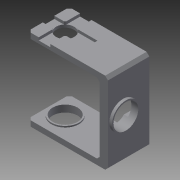
# Autodesk Inventor part: Enlace1
Saved by Autodesk Inventor 2015 (Build 190159000, 159)
## iProperties
Created: 2013-10-22
Part Number: Enlace1
Material: Genérico
Document SubType Name: Modeling
Designer: Gregorio
Density: 1 g/cm^3
Appearance: Valor por defecto
Author: Gregorio
Autodesk Inventor part; units mm, degrees
ref_plane "YZ Plane" through (0, 0, 0) normal (1, 0, 0) x (0, 1, 0)
ref_plane "XZ Plane" through (0, 0, 0) normal (0, 1, 0) x (-1, 0, 0)
ref_plane "XY Plane" through (0, 0, 0) normal (0, 0, 1) x (1, 0, 0)
sketch "Boceto1" plane through (0, 0, 0) normal (0, 1, 0) x (-1, 0, 0)
  line L0 (0, 0) -> (4, 0)
  line L1 (4, 0) -> (4, 58)
  line L2 (4, 58) -> (0, 58)
  line L3 (0, 58) -> (0, 0)
  line L4 (4, 58) -> (59, 58)
  line L5 (59, 58) -> (59, 54)
  line L6 (59, 54) -> (4, 54)
  line L7 (4, 54) -> (4, 58)
  line L8 (4, 0) -> (59, 0)
  line L9 (59, 0) -> (59, 4)
  line L10 (59, 4) -> (4, 4)
  line L11 (4, 4) -> (4, 0)
  dimension "d4" = 58
  dimension "d5" = 55
  dimension "d6" = 4
  dimension "d7" = 55
  dimension "d8" = 4
  dimension "d54" = 4
  constraints: 24 end point, 6 parallel, 3 horizontal, 3 perpendicular
  measures "d4" distance of L0.end L1.end
  measures "d5" distance of L5.end L6.end
  measures "d6" distance of L4.end L5.end
  measures "d7" distance of L10.end L9.end
  measures "d8" distance of L9.end L8.end
  measures "d54" distance of L1.end L2.end
extrude "Extrusión1" add sketch "Boceto1" along normal blind 30
sketch "Boceto3" plane through (-59, 0, 4) normal (0, 0, 1) x (1, 0, 0)
  line L0 (0, 0) -> (0, 30) projected
  circle A0 centre (12, 15) radius 9
  point P0 (59, 0)
  point P1 (0, 15)
  dimension "d19" = 18
  dimension "d20" = 12
  constraints: 1 centre point, 1 horizontal alignment, 1 midpoint
  measures "d19" diameter of A0
  measures "d20" distance from line of L0 A0.centre
extrude "Extrusión2" cut sketch "Boceto3" against normal blind 8 and the other way blind 2
sketch "Boceto5" plane through (0, 0, 58) normal (1, 0, 0) x (0, 0, -1)
  circle A0 centre (29, 11) radius 9
  line L0 (0, 30) -> (58, 30) projected
  line L1 (0, 0) -> (58, 0) projected
  line L2 (58, 0) -> (58, 30) projected
  line L3 (0, 0) -> (0, 30) projected
  point P0 (29, 30)
  point P1 (29, 30)
  dimension "d28" = 18
  dimension "d73" = 11
  constraints: 2 midpoint, 2 vertical alignment, 1 centre point
  measures "d28" diameter of A0
  measures "d73" distance from line of L1 A0.centre
extrude "Extrusión4" cut sketch "Boceto5" against normal blind 20 contours A0
sketch "Boceto6" plane through (-4, 0, 4) normal (-1, 0, 0) x (0, 0, 1)
  circle A0 centre (25, 11) radius 9 projected
  line L0 (0, 30) -> (0, 0) projected
  line L1 (0, 0) -> (50, 0) projected
  line L2 (50, 0) -> (50, 30) projected
  line L3 (0, 30) -> (50, 30) projected
  point P0 (-4, 0)
extrude "Extrusión5" add sketch "Boceto6" along normal blind 4
sketch "Boceto8" plane through (-59, 0, 58) normal (0, 0, 1) x (1, 0, 0)
  circle A0 centre (12, 15) radius 6.5
  line L0 (0, 0) -> (0, 30) projected
  line L1 (0, 9) -> (0, 16)
  point P0 (0, 15)
  dimension "d40" = 13
  dimension "d42" = 12
  constraints: 2 end point, 1 centre point, 1 horizontal alignment, 1 midpoint, 1 point on line
  measures "d40" diameter of A0
  measures "d42" distance from line of L0 A0.centre
extrude "Extrusión7" cut sketch "Boceto8" against normal blind 5
sketch "Boceto9" plane through (-59, 0, 58) normal (0, 0, 1) x (1, 0, 0)
  circle A0 centre (12, 15) radius 6.5 projected
  line L0 (0, 19.15) -> (31.3, 19.15)
  line L1 (31.3, 19.15) -> (31.3, 10.85)
  line L2 (31.3, 10.85) -> (0, 10.85)
  line L3 (0, 10.85) -> (0, 19.15)
  line L4 (0, 0) -> (0, 30) projected
  point P0 (0, 15)
  dimension "d44" = 19.3
  dimension "d45" = 8.3
  constraints: 8 end point, 2 midpoint, 2 parallel, 1 horizontal, 1 horizontal alignment, 1 perpendicular
  measures "d44" distance from line of L1 A0.centre
  measures "d45" distance of L0.end L1.end
sketch "Boceto10" plane through (-59, 0, 58) normal (0, 0, 1) x (1, 0, 0)
  circle A0 centre (12, 15) radius 6.5 projected
  line L0 (0, 0) -> (0, 30) projected
  line L1 (7.85, 33.3) -> (16.15, 33.3)
  line L2 (16.15, 33.3) -> (16.15, -3.3)
  line L3 (16.15, -3.3) -> (7.85, -3.3)
  line L4 (7.85, -3.3) -> (7.85, 33.3)
  point P0 (7.85, 15)
  point P1 (0, 15)
  point P2 (12, 33.3)
  dimension "d48" = 8.3
  dimension "d49" = 36.6
  constraints: 8 end point, 3 midpoint, 2 parallel, 1 horizontal, 1 horizontal alignment, 1 perpendicular, 1 vertical alignment
  measures "d48" distance of L1.start L1.end
  measures "d49" distance of L3.end L1.start
extrude "Extrusión8" cut sketch "Boceto10" against normal blind 2 contours L2 A0 L4 | A0 L4 L1 L2 | L2 L3 L4 A0
extrude "Extrusión9" cut sketch "Boceto9" against normal blind 2 contours A0 L2 L0 | A0 L0 L1 L2 | A0 L2 L3 L0
sketch "Boceto12" plane through (-8, 0, 4) normal (-1, 0, 0) x (0, 0, 1)
  circle A0 centre (25, 11) radius 9 projected
  line L0 (18.85, 4.429) -> (31.15, 4.429)
  line L1 (31.15, 4.429) -> (31.15, 28.029)
  line L2 (31.15, 28.029) -> (18.85, 28.029)
  line L3 (18.85, 28.029) -> (18.85, 4.429)
  point P0 (-4, 0)
  point P1 (25, 4.429)
  dimension "d76" = 12.3
  dimension "d77" = 23.6
  constraints: 8 end point, 2 parallel, 1 horizontal, 1 midpoint, 1 perpendicular, 1 vertical alignment, 2 other
  measures "d76" distance of L2.end L1.end
  measures "d77" distance of L1.end L0.end
extrude "Extrusión11" cut sketch "Boceto12" against normal blind 4 contours L3 A0 L1 L0 | L3 L2 L1 A0
sketch "Boceto13" plane through (0, 0, 58) normal (1, 0, 0) x (0, 0, -1)
  circle A0 centre (29, 11) radius 9 projected
  line L0 (0, 0) -> (58, 0) projected
  line L1 (58, 0) -> (58, 30) projected
  line L2 (0, 30) -> (58, 30) projected
  line L3 (0, 0) -> (0, 30) projected
  circle A1 centre (29, 11) radius 10
  constraints: 1 centre point, 1 coincident
extrude "Extrusión12" cut sketch "Boceto13" against normal blind 1 contours L3 L2 L1 L0
chamfer "Chaflán5" distance 2 angle 45 1 edges at (-1, 15, 58)
sketch "Boceto14" plane through (-8, 0, 4) normal (-1, 0, 0) x (0, 0, 1)
  line L0 (0, 0) -> (0, 30) projected
  line L1 (0, 0) -> (50, 0) projected
  line L2 (50, 30) -> (50, 0) projected
  line L3 (50, 30) -> (0, 30) projected
  line L4 (18.85, 17.571) -> (18.85, 28.029) projected
  line L5 (18.85, 28.029) -> (31.15, 28.029) projected
  line L6 (31.15, 28.029) -> (31.15, 17.571) projected
  arc A0 (18.85, 17.571) -> (31.15, 17.571) centre (25, 11) ccw projected
  point P0 (-4, 0)
extrude "Extrusión13" cut sketch "Boceto14" against normal blind 1
sketch "Boceto16" plane through (-59, 0, 0) normal (0, 0, -1) x (-1, 0, 0)
  line L0 (-58, 30) -> (-58, 0) projected
  line L1 (-58, 0) -> (0, 0) projected
  line L2 (0, 0) -> (0, 30) projected
  line L3 (-58, 30) -> (0, 30) projected
  circle A0 centre (-12, 15) radius 9 projected
  point P0 (-59, 0)
extrude "Extrusión14" add sketch "Boceto16" along normal blind 1
sketch "Boceto18" plane through (-59, 0, 4) normal (0, 0, 1) x (1, 0, 0)
  line L0 (0, 30) -> (52, 30) projected
  line L1 (0, 0) -> (0, 30) projected
  line L2 (0, 0) -> (52, 0) projected
  line L3 (52, 0) -> (52, 30) projected
  circle A0 centre (12, 15) radius 9 projected
  circle A1 centre (12, 15) radius 10
  point P0 (59, 0)
  constraints: 1 centre point, 1 coincident
extrude "Extrusión16" cut sketch "Boceto18" against normal blind 1 contours L0 L3 L2 L1
chamfer "Chaflán8" distance 2 angle 45 2 edges at (-7, 15, 3) (-7, 15, 54)
chamfer "Chaflán9" distance 2 angle 45 1 edges at (-1, 15, -1)
chamfer "Chaflán10" distance 2 angle 45 4 edges at (-59, 30, 1) (-59, 0, 1) (-59, 0, 56) (-59, 30, 56)
sketch "Boceto19" plane through (0, 11, 29) normal (1, 0, 0) x (0, 0, -1)
  circle A0 centre (0, 0) radius 10 projected
  circle A1 centre (0, 0) radius 9 projected
  point P0 (29, -11)
extrude "Extrusión17" add sketch "Boceto19" along normal blind 1
